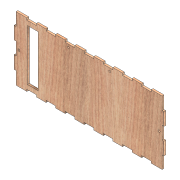
# Autodesk Inventor part: onderplaat elektrobix v2
Saved by Autodesk Inventor 2020.3 (Build 243373000, 373)
## iProperties
Created: 2020-11-25
Part Number: onderplaat elektrobix v2
Material: Wood (Birch)
Document SubType Name: Sheet Metal
Designer: Svend
Density: 0.55 g/cm^3
Sheet Metal Rule: Default_mm
Appearance: Birch - Natural Polished
Author: Svend
Autodesk Inventor part; units mm, degrees
ref_plane "YZ Plane" through (0, 0, 0) normal (1, 0, 0) x (0, 1, 0)
ref_plane "XZ Plane" through (0, 0, 0) normal (0, 1, 0) x (-1, 0, 0)
ref_plane "XY Plane" through (0, 0, 0) normal (0, 0, 1) x (1, 0, 0)
sketch "Sketch1" plane through (0, 0, 0) normal (0, 0, 1) x (1, 0, 0)
  line L0 (-235, 100) -> (235, 100)
  line L1 (235, 100) -> (235, -100)
  line L2 (235, -100) -> (-235, -100)
  line L3 (-235, -100) -> (-235, 100)
  line L4 (-235, 100) -> (235, -100) construction
  line L5 (235, 100) -> (-235, -100) construction
  line L6 (-15, 94) -> (15, 94)
  line L7 (15, 94) -> (15, 100)
  line L8 (15, 100) -> (-15, 100)
  line L9 (-15, 100) -> (-15, 94)
  line L10 (-15, 94) -> (15, 100) construction
  line L11 (15, 94) -> (-15, 100) construction
  line L12 (45, 94) -> (75, 94)
  line L13 (75, 94) -> (75, 100)
  line L14 (75, 100) -> (45, 100)
  line L15 (45, 100) -> (45, 94)
  line L16 (45, 94) -> (75, 100) construction
  line L17 (75, 94) -> (45, 100) construction
  line L18 (105, 94) -> (135, 94)
  line L19 (135, 94) -> (135, 100)
  line L20 (135, 100) -> (105, 100)
  line L21 (105, 100) -> (105, 94)
  line L22 (105, 94) -> (135, 100) construction
  line L23 (135, 94) -> (105, 100) construction
  line L24 (165, 94) -> (195, 94)
  line L25 (195, 94) -> (195, 100)
  line L26 (195, 100) -> (165, 100)
  line L27 (165, 100) -> (165, 94)
  line L28 (165, 94) -> (195, 100) construction
  line L29 (195, 94) -> (165, 100) construction
  line L30 (-75, 94) -> (-45, 94)
  line L31 (-45, 94) -> (-45, 100)
  line L32 (-45, 100) -> (-75, 100)
  line L33 (-75, 100) -> (-75, 94)
  line L34 (-75, 94) -> (-45, 100) construction
  line L35 (-45, 94) -> (-75, 100) construction
  line L36 (-15, 94) -> (15, 94)
  line L37 (15, 94) -> (15, 100)
  line L38 (15, 100) -> (-15, 100)
  line L39 (-15, 100) -> (-15, 94)
  line L40 (-15, 94) -> (15, 100) construction
  line L41 (15, 94) -> (-15, 100) construction
  line L42 (45, 94) -> (75, 94)
  line L43 (75, 94) -> (75, 100)
  line L44 (75, 100) -> (45, 100)
  line L45 (45, 100) -> (45, 94)
  line L46 (45, 94) -> (75, 100) construction
  line L47 (75, 94) -> (45, 100) construction
  line L48 (105, 94) -> (135, 94)
  line L49 (135, 94) -> (135, 100)
  line L50 (135, 100) -> (105, 100)
  line L51 (105, 100) -> (105, 94)
  line L52 (105, 94) -> (135, 100) construction
  line L53 (135, 94) -> (105, 100) construction
  line L54 (-135, 94) -> (-105, 94)
  line L55 (-105, 94) -> (-105, 100)
  line L56 (-105, 100) -> (-135, 100)
  line L57 (-135, 100) -> (-135, 94)
  line L58 (-135, 94) -> (-105, 100) construction
  line L59 (-105, 94) -> (-135, 100) construction
  line L60 (-75, 94) -> (-45, 94)
  line L61 (-45, 94) -> (-45, 100)
  line L62 (-45, 100) -> (-75, 100)
  line L63 (-75, 100) -> (-75, 94)
  line L64 (-75, 94) -> (-45, 100) construction
  line L65 (-45, 94) -> (-75, 100) construction
  line L66 (-15, 94) -> (15, 94)
  line L67 (15, 94) -> (15, 100)
  line L68 (15, 100) -> (-15, 100)
  line L69 (-15, 100) -> (-15, 94)
  line L70 (-15, 94) -> (15, 100) construction
  line L71 (15, 94) -> (-15, 100) construction
  line L72 (45, 94) -> (75, 94)
  line L73 (75, 94) -> (75, 100)
  line L74 (75, 100) -> (45, 100)
  line L75 (45, 100) -> (45, 94)
  line L76 (45, 94) -> (75, 100) construction
  line L77 (75, 94) -> (45, 100) construction
  line L78 (-195, 94) -> (-165, 94)
  line L79 (-165, 94) -> (-165, 100)
  line L80 (-165, 100) -> (-195, 100)
  line L81 (-195, 100) -> (-195, 94)
  line L82 (-195, 94) -> (-165, 100) construction
  line L83 (-165, 94) -> (-195, 100) construction
  line L84 (-135, 94) -> (-105, 94)
  line L85 (-105, 94) -> (-105, 100)
  line L86 (-105, 100) -> (-135, 100)
  line L87 (-135, 100) -> (-135, 94)
  line L88 (-135, 94) -> (-105, 100) construction
  line L89 (-105, 94) -> (-135, 100) construction
  line L90 (-75, 94) -> (-45, 94)
  line L91 (-45, 94) -> (-45, 100)
  line L92 (-45, 100) -> (-75, 100)
  line L93 (-75, 100) -> (-75, 94)
  line L94 (-75, 94) -> (-45, 100) construction
  line L95 (-45, 94) -> (-75, 100) construction
  line L96 (-15, 94) -> (15, 94)
  line L97 (15, 94) -> (15, 100)
  line L98 (15, 100) -> (-15, 100)
  line L99 (-15, 100) -> (-15, 94)
  line L100 (-15, 94) -> (15, 100) construction
  line L101 (15, 94) -> (-15, 100) construction
  line L102 (229, -20) -> (235, -20)
  line L103 (235, -20) -> (235, 20)
  line L104 (235, 20) -> (229, 20)
  line L105 (229, 20) -> (229, -20)
  line L106 (229, -20) -> (235, 20) construction
  line L107 (235, -20) -> (229, 20) construction
  line L108 (235, 100) -> (229, 100)
  line L109 (229, 100) -> (229, 60)
  line L110 (229, 60) -> (235, 60)
  line L111 (235, 60) -> (235, 100)
  line L112 (235, -100) -> (229, -100)
  line L113 (229, -100) -> (229, -60)
  line L114 (229, -60) -> (235, -60)
  line L115 (235, -60) -> (235, -100)
  line L116 (0, 100) -> (0, -100) construction
  line L117 (235, 0) -> (-235, 0) construction
  line L118 (-229, -20) -> (-235, -20)
  line L119 (-235, -20) -> (-235, 20)
  line L120 (-235, 20) -> (-229, 20)
  line L121 (-229, 20) -> (-229, -20)
  line L122 (-229, -20) -> (-235, 20) construction
  line L123 (-235, -20) -> (-229, 20) construction
  line L124 (-235, 100) -> (-229, 100)
  line L125 (-229, 100) -> (-229, 60)
  line L126 (-229, 60) -> (-235, 60)
  line L127 (-235, 60) -> (-235, 100)
  line L128 (-235, -100) -> (-229, -100)
  line L129 (-229, -100) -> (-229, -60)
  line L130 (-229, -60) -> (-235, -60)
  line L131 (-235, -60) -> (-235, -100)
  line L132 (-15, -94) -> (15, -94)
  line L133 (15, -94) -> (15, -100)
  line L134 (15, -100) -> (-15, -100)
  line L135 (-15, -100) -> (-15, -94)
  line L136 (-15, -94) -> (15, -100) construction
  line L137 (15, -94) -> (-15, -100) construction
  line L138 (45, -100) -> (45, -94)
  line L139 (45, -94) -> (75, -94)
  line L140 (75, -100) -> (45, -100)
  line L141 (45, -94) -> (75, -100) construction
  line L142 (75, -94) -> (45, -100) construction
  line L143 (75, -94) -> (75, -100)
  line L144 (105, -100) -> (105, -94)
  line L145 (105, -94) -> (135, -94)
  line L146 (135, -100) -> (105, -100)
  line L147 (105, -94) -> (135, -100) construction
  line L148 (135, -94) -> (105, -100) construction
  line L149 (135, -94) -> (135, -100)
  line L150 (165, -100) -> (165, -94)
  line L151 (165, -94) -> (195, -94)
  line L152 (195, -100) -> (165, -100)
  line L153 (165, -94) -> (195, -100) construction
  line L154 (195, -94) -> (165, -100) construction
  line L155 (195, -94) -> (195, -100)
  line L156 (-75, -100) -> (-75, -94)
  line L157 (-75, -94) -> (-45, -94)
  line L158 (-45, -100) -> (-75, -100)
  line L159 (-75, -94) -> (-45, -100) construction
  line L160 (-45, -94) -> (-75, -100) construction
  line L161 (-45, -94) -> (-45, -100)
  line L162 (-15, -100) -> (-15, -94)
  line L163 (-15, -94) -> (15, -94)
  line L164 (15, -100) -> (-15, -100)
  line L165 (-15, -94) -> (15, -100) construction
  line L166 (15, -94) -> (-15, -100) construction
  line L167 (15, -94) -> (15, -100)
  line L168 (45, -100) -> (45, -94)
  line L169 (45, -94) -> (75, -94)
  line L170 (75, -100) -> (45, -100)
  line L171 (45, -94) -> (75, -100) construction
  line L172 (75, -94) -> (45, -100) construction
  line L173 (75, -94) -> (75, -100)
  line L174 (105, -100) -> (105, -94)
  line L175 (105, -94) -> (135, -94)
  line L176 (135, -100) -> (105, -100)
  line L177 (105, -94) -> (135, -100) construction
  line L178 (135, -94) -> (105, -100) construction
  line L179 (135, -94) -> (135, -100)
  line L180 (-135, -100) -> (-135, -94)
  line L181 (-135, -94) -> (-105, -94)
  line L182 (-105, -100) -> (-135, -100)
  line L183 (-135, -94) -> (-105, -100) construction
  line L184 (-105, -94) -> (-135, -100) construction
  line L185 (-105, -94) -> (-105, -100)
  line L186 (-75, -100) -> (-75, -94)
  line L187 (-75, -94) -> (-45, -94)
  line L188 (-45, -100) -> (-75, -100)
  line L189 (-75, -94) -> (-45, -100) construction
  line L190 (-45, -94) -> (-75, -100) construction
  line L191 (-45, -94) -> (-45, -100)
  line L192 (-15, -100) -> (-15, -94)
  line L193 (-15, -94) -> (15, -94)
  line L194 (15, -100) -> (-15, -100)
  line L195 (-15, -94) -> (15, -100) construction
  line L196 (15, -94) -> (-15, -100) construction
  line L197 (15, -94) -> (15, -100)
  line L198 (45, -100) -> (45, -94)
  line L199 (45, -94) -> (75, -94)
  line L200 (75, -100) -> (45, -100)
  line L201 (45, -94) -> (75, -100) construction
  line L202 (75, -94) -> (45, -100) construction
  line L203 (75, -94) -> (75, -100)
  line L204 (-195, -100) -> (-195, -94)
  line L205 (-195, -94) -> (-165, -94)
  line L206 (-165, -100) -> (-195, -100)
  line L207 (-195, -94) -> (-165, -100) construction
  line L208 (-165, -94) -> (-195, -100) construction
  line L209 (-165, -94) -> (-165, -100)
  line L210 (-135, -100) -> (-135, -94)
  line L211 (-135, -94) -> (-105, -94)
  line L212 (-105, -100) -> (-135, -100)
  line L213 (-135, -94) -> (-105, -100) construction
  line L214 (-105, -94) -> (-135, -100) construction
  line L215 (-105, -94) -> (-105, -100)
  line L216 (-75, -100) -> (-75, -94)
  line L217 (-75, -94) -> (-45, -94)
  line L218 (-45, -100) -> (-75, -100)
  line L219 (-75, -94) -> (-45, -100) construction
  line L220 (-45, -94) -> (-75, -100) construction
  line L221 (-45, -94) -> (-45, -100)
  line L222 (-15, -100) -> (-15, -94)
  line L223 (-15, -94) -> (15, -94)
  line L224 (15, -100) -> (-15, -100)
  line L225 (-15, -94) -> (15, -100) construction
  line L226 (15, -94) -> (-15, -100) construction
  line L227 (15, -94) -> (15, -100)
  circle A0 centre (-65, 85) radius 3
  circle A1 centre (65, 85) radius 3
  line L228 (65, 85) -> (-65, 85) construction
  circle A2 centre (-220, 0) radius 3
  circle A3 centre (220, 0) radius 3
  point P0 (0, 0)
  point P1 (0, 97)
  point P2 (0, 97)
  point P3 (0, 0)
  point P4 (60, 97)
  point P5 (60, 97)
  point P6 (120, 97)
  point P7 (120, 97)
  point P8 (180, 97)
  point P9 (180, 97)
  point P10 (-60, 97)
  point P11 (-60, 97)
  point P12 (0, 97)
  point P13 (0, 97)
  point P14 (60, 97)
  point P15 (60, 97)
  point P16 (120, 97)
  point P17 (120, 97)
  point P18 (-120, 97)
  point P19 (-120, 97)
  point P20 (-60, 97)
  point P21 (-60, 97)
  point P22 (0, 97)
  point P23 (0, 97)
  point P24 (60, 97)
  point P25 (60, 97)
  point P26 (-180, 97)
  point P27 (-180, 97)
  point P28 (-120, 97)
  point P29 (-120, 97)
  point P30 (-60, 97)
  point P31 (-60, 97)
  point P32 (0, 97)
  point P33 (0, 97)
  point P34 (232, 0)
  point P35 (232, 0)
  point P36 (0, 0)
  point P37 (-232, 0)
  point P38 (-232, 0)
  point P39 (0, -97)
  point P40 (60, -100)
  point P41 (60, -97)
  point P42 (120, -100)
  point P43 (120, -97)
  point P44 (180, -100)
  point P45 (180, -97)
  point P46 (-60, -100)
  point P47 (-60, -97)
  point P48 (0, -97)
  point P49 (60, -100)
  point P50 (60, -97)
  point P51 (120, -100)
  point P52 (120, -97)
  point P53 (-120, -100)
  point P54 (-120, -97)
  point P55 (-60, -100)
  point P56 (-60, -97)
  point P57 (0, -97)
  point P58 (60, -100)
  point P59 (60, -97)
  point P60 (-180, -100)
  point P61 (-180, -97)
  point P62 (-120, -100)
  point P63 (-120, -97)
  point P64 (-60, -100)
  point P65 (-60, -97)
  point P66 (0, -97)
  point P67 (0, 85)
  point P68 (0, 100)
  dimension "d0" = 470
  dimension "d1" = 200
  dimension "d2" = 6
  dimension "d3" = 30
  dimension "d6" = 60
  dimension "d9" = 60
  dimension "d12" = 6
  dimension "d13" = 40
  dimension "d14" = 6
  dimension "d15" = 40
  dimension "d16" = 6
  dimension "d17" = 40
  dimension "d20" = 60
  dimension "d23" = 60
  dimension "d26" = 6
  dimension "d27" = 15
  dimension "d28" = 130
  dimension "d29" = 6
  dimension "d30" = 6
  dimension "d31" = 15
  dimension "d32" = 15
  measures "d0" distance of L1.end L2.end
  measures "d1" distance of L0.end L1.end
  measures "d2" distance of L6.end L7.end
  measures "d3" distance of L6.start L6.end
  measures "d6" distance of L6.start L12.start
  measures "d9" distance of L6.start L30.start
  measures "d12" distance of L103.end L104.end
  measures "d13" distance of L104.end L102.start
  measures "d14" distance of L110.end L109.end
  measures "d15" distance of L109.end L108.end
  measures "d16" distance of L113.end L114.end
  measures "d17" distance of L112.end L113.end
  measures "d20" distance of L116.end point (60, -100)
  measures "d23" distance of L116.end point (-60, -100)
  measures "d26" diameter of A1
  measures "d27" distance between parallel lines of L0 L228
  measures "d28" distance of L228.start L228.end
  measures "d29" diameter of A2
  measures "d30" diameter of A3
  measures "d31" distance from line of L3 A2.centre
  measures "d32" distance from line of L103 A3.centre
extrude "Plate1" add sketch "Sketch1" along normal blind 6 contours L0 L81 L78 L79 L57 L54 L55 L33 L30 L31 L9 L6 L7 L15 L12 L13 L21 L18 L19 L27 L24 L25 L109 L110 L1 L104 L105 L102 L114 L113 L2 L155 L151 L150 L149 L145 L144 L143 L139 L138 L133 L132 L135 L161 L157 L156 L185 L181 L180 L209 L205 L204 L129 L130 L3 L118 L121 L120 L126 L125
sketch "Sketch2" plane through (0, 0, 0) normal (0, 0, -1) x (-1, 0, 0)
  line L0 (160, -80) -> (193, -80)
  line L1 (193, -80) -> (193, 80)
  line L2 (193, 80) -> (160, 80)
  line L3 (160, 80) -> (160, -80)
  circle A0 centre (65, 85) radius 3 projected
  circle A1 centre (-65, 85) radius 3 projected
  circle A2 centre (220, 0) radius 3 projected
  circle A3 centre (-220, 0) radius 3 projected
  line L4 (235, -20) -> (229, -20) projected
  line L5 (229, -20) -> (229, 20) projected
  line L6 (229, 20) -> (235, 20) projected
  line L7 (235, 60) -> (235, 20) projected
  line L8 (235, 60) -> (229, 60) projected
  line L9 (229, 60) -> (229, 100) projected
  line L10 (195, 100) -> (229, 100) projected
  line L11 (195, 100) -> (195, 94) projected
  line L12 (195, 94) -> (165, 94) projected
  line L13 (165, 94) -> (165, 100) projected
  line L14 (135, 100) -> (165, 100) projected
  line L15 (135, 100) -> (135, 94) projected
  line L16 (135, 94) -> (105, 94) projected
  line L17 (105, 94) -> (105, 100) projected
  line L18 (75, 100) -> (105, 100) projected
  line L19 (75, 100) -> (75, 94) projected
  line L20 (75, 94) -> (45, 94) projected
  line L21 (45, 94) -> (45, 100) projected
  line L22 (15, 100) -> (45, 100) projected
  line L23 (15, 100) -> (15, 94) projected
  line L24 (15, 94) -> (-15, 94) projected
  line L25 (-15, 94) -> (-15, 100) projected
  line L26 (-45, 100) -> (-15, 100) projected
  line L27 (-45, 100) -> (-45, 94) projected
  line L28 (-45, 94) -> (-75, 94) projected
  line L29 (-75, 94) -> (-75, 100) projected
  line L30 (-105, 100) -> (-75, 100) projected
  line L31 (-105, 100) -> (-105, 94) projected
  line L32 (-105, 94) -> (-135, 94) projected
  line L33 (-135, 94) -> (-135, 100) projected
  line L34 (-165, 100) -> (-135, 100) projected
  line L35 (-165, 100) -> (-165, 94) projected
  line L36 (-165, 94) -> (-195, 94) projected
  line L37 (-195, 94) -> (-195, 100) projected
  line L38 (-229, 100) -> (-195, 100) projected
  line L39 (-229, 100) -> (-229, 60) projected
  line L40 (-229, 60) -> (-235, 60) projected
  line L41 (-235, 20) -> (-235, 60) projected
  line L42 (-235, 20) -> (-229, 20) projected
  line L43 (-229, 20) -> (-229, -20) projected
  line L44 (-229, -20) -> (-235, -20) projected
  line L45 (-235, -60) -> (-235, -20) projected
  line L46 (-235, -60) -> (-229, -60) projected
  line L47 (-229, -60) -> (-229, -100) projected
  line L48 (-195, -100) -> (-229, -100) projected
  line L49 (-195, -100) -> (-195, -94) projected
  line L50 (-195, -94) -> (-165, -94) projected
  line L51 (-165, -94) -> (-165, -100) projected
  line L52 (-135, -100) -> (-165, -100) projected
  line L53 (-135, -100) -> (-135, -94) projected
  line L54 (-135, -94) -> (-105, -94) projected
  line L55 (-105, -94) -> (-105, -100) projected
  line L56 (-75, -100) -> (-105, -100) projected
  line L57 (-75, -100) -> (-75, -94) projected
  line L58 (-75, -94) -> (-45, -94) projected
  line L59 (-45, -94) -> (-45, -100) projected
  line L60 (-15, -100) -> (-45, -100) projected
  line L61 (-15, -100) -> (-15, -94) projected
  line L62 (-15, -94) -> (15, -94) projected
  line L63 (15, -94) -> (15, -100) projected
  line L64 (45, -100) -> (15, -100) projected
  line L65 (45, -100) -> (45, -94) projected
  line L66 (45, -94) -> (75, -94) projected
  line L67 (75, -94) -> (75, -100) projected
  line L68 (105, -100) -> (75, -100) projected
  line L69 (105, -100) -> (105, -94) projected
  line L70 (105, -94) -> (135, -94) projected
  line L71 (135, -94) -> (135, -100) projected
  line L72 (165, -100) -> (135, -100) projected
  line L73 (165, -100) -> (165, -94) projected
  line L74 (165, -94) -> (195, -94) projected
  line L75 (195, -94) -> (195, -100) projected
  line L76 (229, -100) -> (195, -100) projected
  line L77 (229, -100) -> (229, -60) projected
  line L78 (229, -60) -> (235, -60) projected
  line L79 (235, -20) -> (235, -60) projected
  point P0 (0, 0)
  point P1 (193, 0)
  point P2 (229, 0)
  dimension "d34" = 33
  dimension "d35" = 160
  dimension "d36" = 36
  constraints: 8 end point, 2 midpoint, 2 parallel, 1 horizontal, 1 horizontal alignment, 1 perpendicular
  measures "d34" distance of L2.end L1.end
  measures "d35" distance of L1.end L0.end
  measures "d36" distance between parallel lines of L5 L1
extrude "Cut1" cut sketch "Sketch2" against normal blind 6 contours L3 L2 L1 L0
equation "\"d12\" = d2"
equation "\"d15\" = d13"
equation "\"d30\" = d29"
equation "\"d32\" = d31"
equation "\"d37\" = Thickness"
equation "\"d33\" = Thickness"
equation "\"BendRadius\" = Thickness"
equation "\"BendReliefWidth\" = Thickness"
equation "\"BendReliefDepth\" = 0.5 * Thickness"
equation "\"CornerReliefSize\" = 4 * Thickness"
equation "\"MinimumRemnant\" = 2 * Thickness"
equation "\"TransitionRadius\" = BendRadius"
equation "\"JacobiRadiusSize\" = BendRadius"
equation "\"GapSize\" = Thickness"
equation "\"Thickness\" = 6"
body "Solid1"
